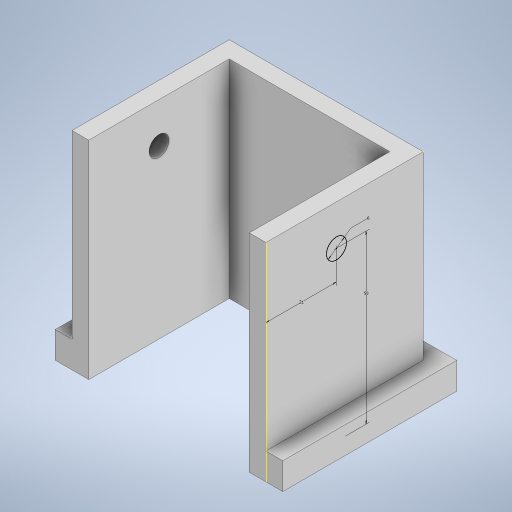
# Autodesk Inventor part: top cam mount v02
Saved by Autodesk Inventor 2023 (Build 270158000, 158)
## iProperties
Created: 2024-07-05
Part Number: top cam mount v02
Material: Generic
Document SubType Name: Modeling
Designer: Akramilab
Density: 1 g/cm^3
Appearance: Default
Author: Akramilab
Autodesk Inventor part; units mm, degrees
ref_plane "YZ Plane" through (0, 0, 0) normal (1, 0, 0) x (0, 1, 0)
ref_plane "XZ Plane" through (0, 0, 0) normal (0, 1, 0) x (-1, 0, 0)
ref_plane "XY Plane" through (0, 0, 0) normal (0, 0, 1) x (1, 0, 0)
sketch "Sketch1" plane through (0, 0, 0) normal (0, 1, 0) x (-1, 0, 0)
  line L0 (0, 0) -> (-58, 0)
  line L1 (-58, 0) -> (-58, 5)
  line L2 (-58, 5) -> (0, 5)
  line L3 (0, 5) -> (0, 0)
  line L4 (0, 5) -> (-5, 5)
  line L5 (-5, 5) -> (-5, 47)
  line L6 (-5, 47) -> (0, 47)
  line L7 (0, 47) -> (0, 5)
  line L8 (-58, 5) -> (-53, 5)
  line L9 (-53, 5) -> (-53, 47)
  line L10 (-53, 47) -> (-58, 47)
  line L11 (-58, 47) -> (-58, 5)
  dimension "d0" = 58
  dimension "d1" = 5
  dimension "d2" = 5
  dimension "d3" = 42
  dimension "d4" = 5
  dimension "d5" = 42
  constraints: 24 end point, 6 parallel, 3 horizontal, 3 perpendicular
  measures "d0" distance of L1.end L2.end
  measures "d1" distance of L0.end L1.end
  measures "d2" distance of L5.end L6.end
  measures "d3" distance of L4.end L5.end
  measures "d4" distance of L10.end L9.end
  measures "d5" distance of L9.end L8.end
extrude "Extrusion1" add sketch "Sketch1" against normal blind 62
sketch "Sketch2" plane through (58, 0, 47) normal (1, 0, 0) x (0, 0, -1)
  line L0 (0, 0) -> (0, -62) projected
  line L1 (47, -62) -> (0, -62) projected
  circle A0 centre (21, -12) radius 3
  point P0 (47, 0)
  point P1 (23.5, -62)
  dimension "d8" = 21
  dimension "d9" = 50
  dimension "d10" = 6
  constraints: 1 centre point, 1 coincident, 1 midpoint
  measures "d8" distance from line of L0 point (21, -12)
  measures "d9" vertical distance of point (21, -12) point (23.5, -62)
  measures "d10" diameter of A0
sketch "Sketch3" plane through (0, -62, 0) normal (0, -1, 0) x (1, 0, 0)
  line L0 (53, 47) -> (58, 47) projected
  line L1 (58, 47) -> (63, 47)
  line L2 (63, 47) -> (63, 0)
  line L3 (63, 0) -> (58, 0)
  line L4 (58, 0) -> (58, 47)
  line L5 (0, 0) -> (0, 47) projected
  line L6 (0, 47) -> (-5, 47)
  line L7 (-5, 47) -> (-5, 0)
  line L8 (-5, 0) -> (0, 0)
  line L9 (0, 0) -> (0, 47)
  line L10 (63, 0) -> (-5, 0)
  line L11 (-5, 0) -> (-5, -5)
  line L12 (-5, -5) -> (63, -5)
  line L13 (63, -5) -> (63, 0)
  dimension "d13" = 5
  dimension "d14" = 5
  dimension "d15" = 5
  constraints: 24 end point, 6 parallel, 3 horizontal, 3 perpendicular, 1 point on line
  measures "d13" distance of L2.end L3.end
  measures "d14" distance of L7.end L8.end
  measures "d15" distance of L12.end L2.end
extrude "Extrusion3" add sketch "Sketch3" against normal blind 8
sketch "Sketch4" plane through (0, -62, 0) normal (0, -1, 0) x (1, 0, 0)
  line L0 (58, 47) -> (58, 0) projected
  line L1 (63, 47) -> (53, 47) projected
  line L2 (0, 0) -> (0, 47) projected
  line L3 (5, 47) -> (-5, 47) projected
  circle A0 centre (58, 37) radius 2.5
  circle A1 centre (0, 37) radius 2.5
  line L4 (58, 0) -> (0, 0) projected
  circle A2 centre (16.5, 0) radius 2.5
  circle A3 centre (41.5, 0) radius 2.5
  point P0 (29, 0)
  dimension "d18" = 10
  dimension "d19" = 10
  dimension "d20" = 5
  dimension "d21" = 5
  dimension "d29" = 5
  dimension "d30" = 5
  constraints: 4 centre point, 4 point on line, 2 coincident
  measures "d18" distance from line of L1 point (58, 37)
  measures "d19" distance from line of L3 point (0, 37)
  measures "d20" diameter of A0
  measures "d21" diameter of A1
  measures "d29" diameter of A2
  measures "d30" diameter of A3
sketch "Sketch5" plane through (0, 0, 0) normal (-1, 0, 0) x (0, 0, 1)
  circle A0 centre (26, -12) radius 3 projected
  circle A1 centre (26, -12) radius 3
  point P0 (0, 0)
  constraints: 2 coincident, 1 centre point, 1 concentric
extrude "Extrusion5" cut sketch "Sketch5" against normal blind 5
extrude "Extrusion6" cut sketch "Sketch4" against normal blind 5
equation "\"d4\" = d2"
equation "\"d5\" = d3"
equation "\"d14\" = d13"
equation "\"d15\" = d13"
equation "\"d19\" = d18"
equation "\"d21\" = d20"
equation "\"d29\" = d20"
equation "\"d30\" = d20"
body "Solid1"
